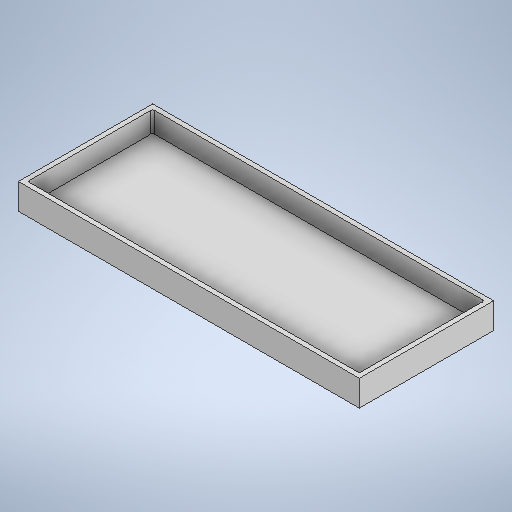
# Autodesk Inventor part: Shelf V2
Saved by Autodesk Inventor 2025 (Build 290162000, 162)
## iProperties
Created: 2025-06-11
Part Number: Shelf V2
Material: Generic
Document SubType Name: Modeling
Designer: Caleb Fangmeier
Density: 1 g/cm^3
Appearance: Default
Author: Caleb Fangmeier
Autodesk Inventor part; units mm, degrees
ref_plane "YZ Plane" through (0, 0, 0) normal (1, 0, 0) x (0, 1, 0)
ref_plane "XZ Plane" through (0, 0, 0) normal (0, 1, 0) x (-1, 0, 0)
ref_plane "XY Plane" through (0, 0, 0) normal (0, 0, 1) x (1, 0, 0)
sketch "Sketch1" plane through (0, 0, 0) normal (0, 1, 0) x (-1, 0, 0)
  line L0 (-165, 65) -> (165, 65)
  line L1 (165, 65) -> (165, -65)
  line L2 (165, -65) -> (-165, -65)
  line L3 (-165, -65) -> (-165, 65)
  line L4 (-165, 65) -> (165, -65) construction
  line L5 (165, 65) -> (-165, -65) construction
  point P0 (0, 0)
  dimension "d0" = 330
  dimension "d1" = 130
  constraints: 12 end point, 2 midpoint, 2 parallel, 1 horizontal, 1 perpendicular
  measures "d0" distance of L1.end L2.end
  measures "d1" distance of L0.end L1.end
extrude "Extrusion1" add sketch "Sketch1" along normal blind 25
sketch "Sketch2" plane through (0, 25, 0) normal (0, 1, 0) x (1, 0, 0)
  line L0 (160.5, -60.5) -> (-160.5, -60.5)
  line L1 (-160.5, -60.5) -> (-160.5, 60.5)
  line L2 (-160.5, 60.5) -> (160.5, 60.5)
  line L3 (160.5, 60.5) -> (160.5, -60.5)
  line L4 (160.5, -60.5) -> (-160.5, 60.5) construction
  line L5 (-160.5, -60.5) -> (160.5, 60.5) construction
  point P0 (0, 0)
  dimension "d4" = 321
  dimension "d5" = 121
  constraints: 12 end point, 2 midpoint, 2 parallel, 1 horizontal, 1 perpendicular
  measures "d4" distance of L1.end L2.end
  measures "d5" distance of L0.end L1.end
extrude "Extrusion2" cut sketch "Sketch2" against normal blind 20
fillet "Fillet1" radius 2 4 edges at (-160.5, 15, -60.5) (160.5, 15, -60.5) (-160.5, 15, 60.5) (160.5, 15, 60.5)
body "Solid1"
